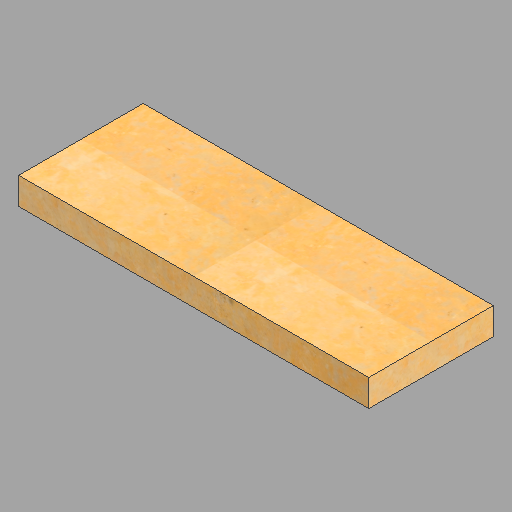
# Autodesk Inventor part: typ
Saved by Autodesk Inventor 2023 (Build 270158030, 158C)
## iProperties
RuleStatus: InUse
Created: 2022-06-16
Part Number: typ
Material: Granite, Cut, Polished
Document SubType Name: Modeling
Designer: awelt
Mass: 170255 g
Surface Area: 16051.6 cm^2
Volume: 63057.4 cm^3
Density: 2.7 g/cm^3
Appearance: Amber Select
AfterDocSave0: Convert in3 volume to ft3
in3 to ft3: 0.0
TEST: 0.001
Author: awelt
Autodesk Inventor part; units mm, degrees
ref_plane "YZ Plane" through (0, 0, 0) normal (1, 0, 0) x (0, 1, 0)
ref_plane "XZ Plane" through (0, 0, 0) normal (0, 1, 0) x (-1, 0, 0)
ref_plane "XY Plane" through (0, 0, 0) normal (0, 0, 1) x (1, 0, 0)
sketch "Sketch1" plane through (0, 0, 0) normal (0, 1, 0) x (-1, 0, 0)
  line L0 (0, 0) -> (-1320.8, 0)
  line L1 (-1320.8, 0) -> (-1320.8, -469.9)
  line L2 (-1320.8, -469.9) -> (0, -469.9)
  line L3 (0, -469.9) -> (0, 0)
  dimension "d0" = 1320.8
  dimension "d1" = 469.9
  constraints: 8 end point, 2 parallel, 1 horizontal, 1 perpendicular
  measures "d0" distance of L2.end L1.end
  measures "d1" distance of L1.end L0.end
extrude "Extrusion1" add sketch "Sketch1" along normal blind 101.6
body "Solid1"
